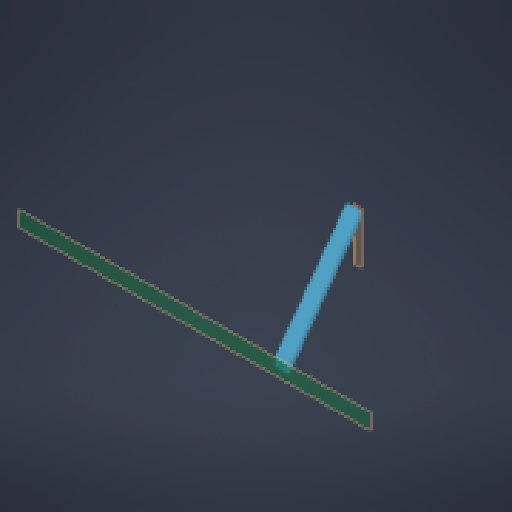
# Autodesk Inventor part: Eyelids
Saved by Autodesk Inventor 2027 (Build 310192000, 192)
## iProperties
Created: 2026-08-07
Part Number: Eyelids
Material: Generic
Document SubType Name: Modeling
Designer: lucas
Density: 1 g/cm^3
Appearance: Default
Author: lucas
Autodesk Inventor part; units mm, degrees
ref_plane "YZ Plane" through (0, 0, 0) normal (1, 0, 0) x (0, 1, 0)
ref_plane "XZ Plane" through (0, 0, 0) normal (0, 1, 0) x (-1, 0, 0)
ref_plane "XY Plane" through (0, 0, 0) normal (0, 0, 1) x (1, 0, 0)
ref_plane "Work Plane1" through (0, 0, 0) normal (0, 0, 1) x (1, 0, 0)
sketch "Sketch1" plane through (0, 0, 0) normal (0, 0, 1) x (1, 0, 0)
  line L0 (50.8, 330.2) -> (-50.8, 330.2)
  line L1 (-50.8, 330.2) -> (-50.8, 279.4)
  line L2 (-50.8, 279.4) -> (50.8, 279.4)
  line L3 (50.8, 279.4) -> (50.8, 330.2)
  point P0 (0, 0)
  dimension "d0" = 50.8
  dimension "d1" = 101.6
  constraints: 8 end point, 2 parallel, 1 horizontal, 1 perpendicular, 1 other
  measures "d0" distance of L0.end L1.end
  measures "d1" distance of L1.end L2.end
ref_plane "Work Plane2" through (-254, -50.8, 863.6) normal (0, 0, -1) x (1, 0, 0)
sketch "Sketch2" plane through (-254, -50.8, 863.6) normal (0, 0, -1) x (1, 0, 0)
  line L0 (1117.6, -50.8) -> (-1117.6, -50.8) projected
  line L1 (662.9873, -50.8) -> (662.9873, 0) projected
  line L2 (662.9873, -50.8) -> (561.3873, -50.8)
  line L3 (561.3873, -50.8) -> (561.3873, 0)
  line L4 (561.3873, 0) -> (662.9873, 0)
  line L5 (662.9873, 0) -> (662.9873, -50.8)
  point P0 (254, -50.8)
  dimension "d2" = 101.6
  constraints: 8 end point, 2 parallel, 1 coincident, 1 horizontal, 1 perpendicular
  measures "d2" distance of L3.end L4.end
loft "Loft1" add profiles "Sketch1", "Sketch2"
body "Solid1"
